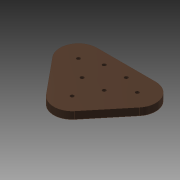
# Autodesk Inventor part: Arm_Base-SquareBar-Rev3-2
Saved by Autodesk Inventor 2015 (Build 190159000, 159)
## iProperties
Created: 2017-03-01
Part Number: Arm_Base-SquareBar-Rev3-2
Material: Bronze, Cast
Document SubType Name: Modeling
Designer: Guy
Density: 8.87 g/cm^3
Appearance: Bronze - Satin
Mass: 790.961 g
Surface Area: 225.637 cm^2
Volume: 89.1726 cm^3
Author: Guy
Autodesk Inventor part; units mm, degrees
ref_plane "YZ Plane" through (0, 0, 0) normal (1, 0, 0) x (0, 1, 0)
ref_plane "XZ Plane" through (0, 0, 0) normal (0, 1, 0) x (-1, 0, 0)
ref_plane "XY Plane" through (0, 0, 0) normal (0, 0, 1) x (1, 0, 0)
sketch "Sketch1" plane through (0, 0, 0) normal (0, 0, 1) x (1, 0, 0)
  circle A0 centre (0, 0) radius 25
  circle A1 centre (40, 48.6) radius 25
  circle A2 centre (-40, 48.6) radius 25
  line L0 (-40, 73.6) -> (40, 73.6)
  line L1 (59.3028, 32.7129) -> (19.3028, -15.8871)
  line L2 (-19.3028, -15.8871) -> (-59.3028, 32.7129)
  dimension "d0" = 50
  dimension "d1" = 50
  dimension "d2" = 50
  dimension "d3" = 40
  dimension "d4" = 40
  dimension "d5" = 48.6
  dimension "d6" = 48.6
  constraints: 6 end point, 6 point on circle, 6 tangent, 3 centre point, 1 coincident
  measures "d0" diameter of A1
  measures "d1" diameter of A0
  measures "d2" diameter of A2
  measures "d3" horizontal distance of point (0, 0) A2.centre
  measures "d4" horizontal distance of point (0, 0) A1.centre
  measures "d5" vertical distance of point (0, 0) A2.centre
  measures "d6" vertical distance of point (0, 0) A1.centre
extrude "Extrusion1" add sketch "Sketch1" along normal blind 10
sketch "Sketch2" plane through (0, 0, 10) normal (0, 0, 1) x (1, 0, 0)
  arc A0 (-40, 73.6) -> (-59.3028, 32.7129) centre (-40, 48.6) ccw projected
  line L0 (-59.3028, 32.7129) -> (-19.3028, -15.8871) projected
  arc A1 (-19.3028, -15.8871) -> (19.3028, -15.8871) centre (0, 0) ccw projected
  line L1 (19.3028, -15.8871) -> (59.3028, 32.7129) projected
  arc A2 (59.3028, 32.7129) -> (40, 73.6) centre (40, 48.6) ccw projected
  line L2 (40, 73.6) -> (-40, 73.6) projected
  circle A3 centre (40, 48.6) radius 2.5
  circle A4 centre (0, 0) radius 2.5
  circle A5 centre (-40, 48.6) radius 2.5
  dimension "d10" = 5
  dimension "d11" = 5
  dimension "d12" = 5
  constraints: 3 centre point, 3 coincident
  measures "d10" diameter of A3
  measures "d11" diameter of A4
  measures "d12" diameter of A5
extrude "Extrusion2" cut sketch "Sketch2" against normal up to next contours A3 | A4 | A5
sketch "Sketch3" plane through (0, 0, 10) normal (0, 0, 1) x (1, 0, 0)
  circle A0 centre (-15, 58.6) radius 2.5
  circle A1 centre (15, 58.6) radius 2.5
  circle A2 centre (-15, 28.6) radius 2.5
  circle A3 centre (15, 28.6) radius 2.5
  circle A4 centre (0, 0) radius 2.5 projected
  circle A5 centre (40, 48.6) radius 2.5 projected
  circle A6 centre (-40, 48.6) radius 2.5 projected
  arc A7 (-40, 73.6) -> (-59.3028, 32.7129) centre (-40, 48.6) ccw projected
  line L0 (-59.3028, 32.7129) -> (-19.3028, -15.8871) projected
  arc A8 (-19.3028, -15.8871) -> (19.3028, -15.8871) centre (0, 0) ccw projected
  line L1 (19.3028, -15.8871) -> (59.3028, 32.7129) projected
  arc A9 (59.3028, 32.7129) -> (40, 73.6) centre (40, 48.6) ccw projected
  line L2 (40, 73.6) -> (-40, 73.6) projected
  dimension "d15" = 5
  dimension "d16" = 5
  dimension "d17" = 5
  dimension "d18" = 5
  dimension "d19" = 30
  dimension "d20" = 30
  dimension "d21" = 30
  dimension "d22" = 30
  dimension "d23" = 15
  dimension "d24" = 15
  dimension "d25" = 15
  dimension "d26" = 15
  constraints: 4 centre point
  measures "d15" diameter of A0
  measures "d16" diameter of A1
  measures "d17" diameter of A2
  measures "d18" diameter of A3
  measures "d19" distance of A1.centre A0.centre
  measures "d20" distance of A3.centre A2.centre
  measures "d21" distance of A3.centre A1.centre
  measures "d22" distance of A2.centre A0.centre
  measures "d23" horizontal distance of A3.centre point (0, 0)
  measures "d24" horizontal distance of point (0, 0) A1.centre
  measures "d25" distance from line of A0.centre L2
  measures "d26" distance from line of L2 A1.centre
extrude "Extrusion3" cut sketch "Sketch3" against normal up to next contours A0 | A1 | A2 | A3
body "Solid1"
